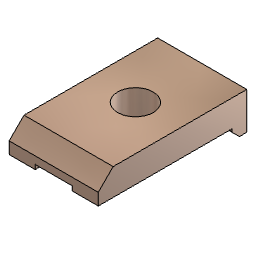
CY7 diode clamp CAM v2 (Autodesk Fusion 360 archive; units mm, degrees)
design "CY7 diode clamp"
Autodesk Fusion 360 part; units mm, degrees
sketch "Sketch1" plane through (0, 0, 0) normal (0, 1, 0) x (1, 0, 0)
  line L0 (-3, 4.5) -> (3, 4.5)
  line L1 (3, 4.5) -> (3, -5.5)
  line L2 (3, -5.5) -> (-3, -5.5)
  line L3 (-3, -5.5) -> (-3, 4.5)
  line L4 (-1.25, -5.5) -> (-1.25, -2.5)
  arc A0 (1.25, -2.5) -> (-1.25, -2.5) centre (0, -2.5) ccw
  line L5 (1.25, -2.5) -> (1.25, -5.5)
  line L6 (-3, 3.5) -> (3, 3.5)
  line L7 (0, 0) -> (0, -2.5) construction
  dimension "d2" = 2.5
  dimension "d3" = 3
  dimension "d4" = 1
  dimension "d5" = 10
  dimension "d6" = 2.5
  dimension "d7" = 6
  constraint horizontal L0
  constraint vertical L1
  constraint horizontal L2
  constraint vertical L3
  constraint coincident L2 L4.start
  constraint perpendicular L2 L4
  constraint tangent L4 A0
  constraint coincident L2 L5.end
  constraint tangent A0 L5
  constraint perpendicular L2 L5
  constraint coincident L3 L6.start
  constraint coincident L1 L6.end
  constraint perpendicular L1 L6
  constraint coincident L7.start origin
  constraint vertical L7.start A0.centre
  constraint coincident A0.centre L7.end
  constraint symmetric L1 L3 L7
  measures "d2" distance of L4 L5
  measures "d3" distance of L2 A0.centre
  measures "d4" distance of L0 L6
  measures "d5" distance of L0 L2
  measures "d6" distance of A0.centre L7.start
  measures "d7" distance of L1 L3
extrude "Extrude1" add sketch "Sketch1" along normal blind 2.5
extrude "Extrude2" cut sketch "Sketch1" along normal blind 0.7 contours L1 L2 L3 L4 A0 L5 L6 | L2 L4 A0 L5
extrude "Extrude3" cut sketch "Sketch1" along normal blind 1 contours L2 L4 A0 L5
hole "Hole1" at (0, 0, 0) direction (0, 1, 0) diameter 2.4 depth 5 tip angle 118
chamfer "Chamfer1" distance 0.5 angle 45 1 edges at (0, 0, -3.5)
chamfer "Chamfer2" distance 1 angle 45 1 edges at (0, 2.5, 5.5)
